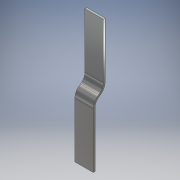
# Autodesk Inventor part: SolarPanel_CellJumper
Saved by Autodesk Inventor 2018 (Build 220112000, 112)
## iProperties
Created: 2020-02-13
Part Number: SolarPanel_CellJumper
Material: Nickel-Copper Alloy 400
Document SubType Name: Modeling
Designer: Bradley
Density: 8.83 g/cm^3
Appearance: Chrome - Polished
Author: Bradley
Autodesk Inventor part; units mm, degrees
ref_plane "YZ Plane" through (0, 0, 0) normal (1, 0, 0) x (0, 1, 0)
ref_plane "XZ Plane" through (0, 0, 0) normal (0, 1, 0) x (-1, 0, 0)
ref_plane "XY Plane" through (0, 0, 0) normal (0, 0, 1) x (1, 0, 0)
sketch "Sketch1" plane through (0, 0, 0) normal (1, 0, 0) x (0, 1, 0)
  line L0 (0, 0) -> (0, -6)
  arc A0 (-0.5, -6.866) -> (0, -6) centre (-1, -6) ccw
  arc A1 (-0.5, -6.866) -> (-1.1, -7.9053) centre (0.1, -7.9053) ccw
  line L1 (-1.1, -7.9053) -> (-1.1, -13.9053)
  line L2 (-1.1, -13.9053) -> (-0.9, -13.9053)
  line L3 (-0.9, -13.9053) -> (-0.9, -7.9053)
  arc A2 (-0.4, -7.0392) -> (-0.9, -7.9053) centre (0.1, -7.9053) ccw
  arc A3 (-0.4, -7.0392) -> (0.2, -6) centre (-1, -6) ccw
  line L4 (0.2, -6) -> (0.2, 0)
  line L5 (0.2, 0) -> (0, 0)
  dimension "d0" = 0.2
  dimension "d1" = 6
  dimension "d2" = 6
  dimension "d3" = 1.1
  dimension "d4" = 1
  constraints: 12 end point, 8 point on circle, 5 tangent, 4 centre point, 3 parallel, 3 perpendicular, 2 concentric, 2 equal radius, 1 vertical
  measures "d0" distance of L4.end L0.start
  measures "d1" distance of L0.start L0.end
  measures "d2" distance of L2.end L3.end
  measures "d3" distance between parallel lines of L1 L0
  measures "d4" radius of A0
extrude "Extrusion1" add sketch "Sketch1" along normal mid plane 2
body "Solid1"
